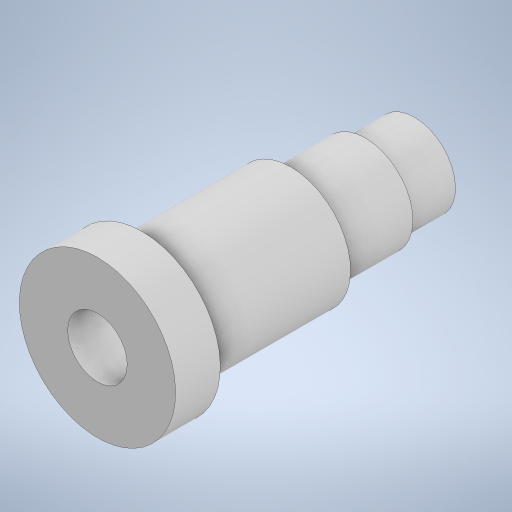
# Autodesk Inventor part: A-2.103-B
Saved by Autodesk Inventor 2023 (Build 270158000, 158)
## iProperties
Created: 2023-07-28
Part Number: A-2.103-B
Material: Generic
Document SubType Name: Modeling
Designer: Graeme
Density: 1 g/cm^3
Appearance: Default
Author: Graeme
Autodesk Inventor part; units mm, degrees
ref_plane "YZ Plane" through (0, 0, 0) normal (1, 0, 0) x (0, 1, 0)
ref_plane "XZ Plane" through (0, 0, 0) normal (0, 1, 0) x (-1, 0, 0)
ref_plane "XY Plane" through (0, 0, 0) normal (0, 0, 1) x (1, 0, 0)
sketch "Sketch1" plane through (0, 0, 0) normal (1, 0, 0) x (0, 1, 0)
  line L0 (0, 12.6765) -> (0, -12.6765)
  line L1 (0, 0) -> (2, 0)
  line L2 (2, 0) -> (2, 10)
  line L3 (2, 10) -> (5.25, 10)
  line L4 (5.25, 10) -> (5.25, 7)
  line L5 (5.25, 7) -> (4, 7)
  line L6 (4, 7) -> (4, -3)
  line L7 (4, -3) -> (3.19, -3)
  line L8 (3.19, -3) -> (3.19, -8)
  line L9 (3.19, -8) -> (2.75, -8)
  line L10 (2.75, -8) -> (2.75, -11.3)
  line L11 (2.75, -11.3) -> (0, -11.3)
  line L12 (0, -11.3) -> (0, 0)
  line L13 (2.75, -18.5) -> (0, -18.5) construction
  point P0 (2, 5)
  dimension "d0" = 4
  dimension "d1" = 3
  dimension "d2" = 10
  dimension "d3" = 10.5
  dimension "d4" = 8
  dimension "d5" = 6.38
  dimension "d6" = 5.5
  dimension "d7" = 28.5
  dimension "d8" = 10.5
  dimension "d9" = 21.3
  dimension "d10" = 13
  constraints: 28 end point, 10 perpendicular, 2 horizontal, 2 midpoint, 1 coincident, 1 collinear, 1 point on line, 1 vertical
  measures "d0" diameter of point (2, 5) L0
  measures "d1" distance of L3.end L4.end
  measures "d2" distance of L1.end L2.end
  measures "d3" diameter of L4 L0
  measures "d4" diameter of L6 L0
  measures "d5" diameter of L8 L0
  measures "d6" diameter of L10 L0
  measures "d7" distance between parallel lines of L13 L3
  measures "d8" distance between parallel lines of L9 L13
  measures "d9" distance between parallel lines of L11 L3
  measures "d10" distance between parallel lines of L7 L3
revolve "Revolution1" add sketch "Sketch1" angle 360 about axis through (0, 0, 12.6765) along (0, 0, -1)
body "Solid1"
